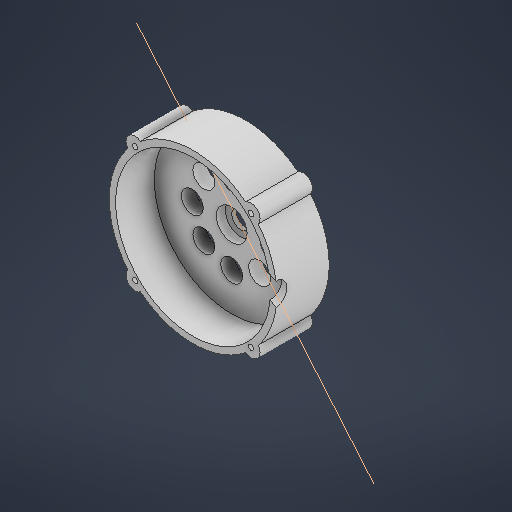
# Autodesk Inventor part: Case Part 1 - V3
Saved by Autodesk Inventor 2025.3 (Build 293356030, 356C)
## iProperties
Created: 2025-09-18
Part Number: Case Part 1 - V3
Material: Generic
Document SubType Name: Modeling
Designer: yo
Density: 1 g/cm^3
Appearance: Default
Author: yo
Autodesk Inventor part; units mm, degrees
ref_plane "YZ Plane" through (0, 0, 0) normal (1, 0, 0) x (0, 1, 0)
ref_plane "XZ Plane" through (0, 0, 0) normal (0, 1, 0) x (-1, 0, 0)
sketch "Sketch1" plane through (0, 0, 0) normal (0, 0, 1) x (1, 0, 0)
  circle A0 centre (0, 0) radius 5
  circle A1 centre (0, 0) radius 8.45
  circle A2 centre (0, 0) radius 42.5
  circle A3 centre (0, 0) radius 45 construction
  circle A4 centre (-31.8198, 31.8198) radius 1.45
  arc A5 (-28.0933, 35.1535) -> (-35.1535, 28.0933) centre (-31.8198, 31.8198) ccw
  arc A6 (-35.1535, -28.0933) -> (-28.0933, -35.1535) centre (-31.8198, -31.8198) ccw
  circle A7 centre (-31.8198, -31.8198) radius 1.45
  arc A8 (28.0933, -35.1535) -> (35.1535, -28.0933) centre (31.8198, -31.8198) ccw
  circle A9 centre (31.8198, -31.8198) radius 1.45
  arc A10 (35.1535, 28.0933) -> (28.0933, 35.1535) centre (31.8198, 31.8198) ccw
  circle A11 centre (31.8198, 31.8198) radius 1.45
  line L0 (-31.8198, 31.8198) -> (31.8198, 31.8198) construction
  arc A12 (28.841, 35.8357) -> (-28.841, 35.8357) centre (0, 0) ccw
  arc A13 (-35.8357, 28.841) -> (-35.8357, -28.841) centre (0, 0) ccw
  arc A14 (-28.841, -35.8357) -> (28.841, -35.8357) centre (0, 0) ccw
  arc A15 (35.8357, -28.841) -> (35.8357, 28.841) centre (0, 0) ccw
  point P0 (0, -46)
  point P1 (0, 46)
  dimension "d2" = 10
  dimension "d3" = 16.9
  dimension "d4" = 85
  dimension "d5" = 90
  dimension "d6" = 2.9
  dimension "d7" = 5
  dimension "d8" = 360
  dimension "d9" = 92
  constraints: 29 point on circle, 16 centre point, 10 coincident, 3 concentric, 2 end point, 1 horizontal, 25 other
  measures "d2" diameter of A0
  measures "d3" diameter of A1
  measures "d4" diameter of A2
  measures "d5" diameter of A3
  measures "d6" diameter of A4
  measures "d7" radius of A5
  measures "d9" distance of point (0, -46) point (0, 46)
extrude "Extrusion1" add sketch "Sketch1" along normal blind 2.5 contours A1
extrude "Extrusion2" add sketch "Sketch1" along normal blind 7.5 contours A2
extrude "Extrusion3" add sketch "Sketch1" along normal blind 28.75 contours A12 A10 A15 A8 A14 A6 A13 A5
sketch "Sketch2" plane through (0, 0, 28.75) normal (0, 0, 1) x (1, 0, 0)
  arc A0 (35.8357, -28.841) -> (35.8357, 28.841) centre (0, 0) ccw construction
  line L0 (46, 0) -> (46, -31.8198) construction
  point P0 (31.8198, -31.8198)
  constraints: 2 end point, 1 horizontal alignment, 1 point on circle, 1 tangent, 1 vertical
ref_plane "Work Plane1" through (46, 0, 28.75) normal (0.9659, 0, 0.2588) x (0, -1, 0)
sketch "Sketch3" plane through (46, 0, 28.75) normal (0.9659, 0, 0.2588) x (0, -1, 0)
  ellipse E0 centre (0, -11.9057) end of major axis (-46, -11.9057) minor radius 11.9057 (28.841, -2.6307) -> (-28.841, -2.6307) ccw projected
  line L0 (0, 0) -> (0, -11.9057) construction
  point P0 (0, 15.8647)
  constraints: 2 end point, 1 vertical, 2 other
ref_plane "Work Plane2" through (46, 0, 28.75) normal (0.8365, -0.5, 0.2241) x (-0.2588, 0, 0.9659)
sketch "Sketch4" plane through (46, 0, 28.75) normal (0.8365, -0.5, 0.2241) x (-0.2588, 0, 0.9659)
  circle A0 centre (0, 0) radius 5.325
  point P0 (-15.8647, 25.9368)
  dimension "d18" = 10.65
  constraints: 1 centre point, 1 coincident
  measures "d18" diameter of A0
extrude "Extrusion4" cut sketch "Sketch4" along normal mid plane 30
sketch "Sketch5" plane through (0, 0, 7.5) normal (0, 0, 1) x (1, 0, 0)
  circle A0 centre (0, 21.65) radius 6
  line L0 (0, 21.65) -> (0, 0)
  circle A1 centre (-15.3089, 15.3089) radius 6
  circle A2 centre (-21.65, 0) radius 6
  circle A3 centre (-15.3089, -15.3089) radius 6
  circle A4 centre (0, -21.65) radius 6
  circle A5 centre (15.3089, -15.3089) radius 6
  circle A6 centre (21.65, 0) radius 6
  circle A7 centre (15.3089, 15.3089) radius 6
  dimension "d21" = 12
  dimension "d22" = 21.65
  dimension "d25" = 360
  constraints: 8 centre point, 2 end point, 1 vertical, 1 vertical alignment, 17 other
  measures "d21" diameter of A0
  measures "d22" distance of L0.start L0.end
extrude "Extrusion5" cut sketch "Sketch5" against normal through all
body "Solid1"
